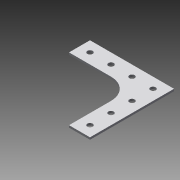
# Autodesk Inventor part: Gusset
Saved by Autodesk Inventor 2015 (Build 190159000, 159)
## iProperties
Created: 2015-01-30
Part Number: Gusset
Material: Generic
Document SubType Name: Modeling
Designer: chapale16
Density: 1 g/cm^3
Appearance: Default
Author: chapale16
Autodesk Inventor part; units mm, degrees
ref_plane "YZ Plane" through (0, 0, 0) normal (1, 0, 0) x (0, 1, 0)
ref_plane "XZ Plane" through (0, 0, 0) normal (0, 1, 0) x (-1, 0, 0)
ref_plane "XY Plane" through (0, 0, 0) normal (0, 0, 1) x (1, 0, 0)
sketch "Sketch1" plane through (0, 0, 0) normal (0, 1, 0) x (-1, 0, 0)
  line L0 (0, 0) -> (0, 101.6)
  line L1 (0, 101.6) -> (25.4, 101.6)
  line L2 (0, 0) -> (101.6, 0)
  line L3 (101.6, 0) -> (101.6, 25.4)
  line L4 (50.8, 25.4) -> (101.6, 25.4)
  line L5 (25.4, 50.8) -> (25.4, 101.6)
  arc A0 (25.4, 28.575) -> (28.575, 25.4) centre (28.575, 28.575) ccw
  arc A1 (25.4, 50.8) -> (50.8, 25.4) centre (50.8, 50.8) ccw
  dimension "d0" = 101.6
  dimension "d1" = 25.4
  dimension "d2" = 101.6
  dimension "d3" = 25.4
  dimension "d4" = 3.175
  dimension "d5" = 25.4
  constraints: 12 end point, 4 perpendicular, 4 point on circle, 4 tangent, 2 centre point, 2 point on line, 1 horizontal, 1 vertical
  measures "d0" distance of L0.start L0.end
  measures "d1" distance of L0.end L1.end
  measures "d2" distance of L0.start L2.end
  measures "d3" distance of L2.end L3.end
  measures "d4" radius of A0
  measures "d5" radius of A1
extrude "Extrusion1" add sketch "Sketch1" along normal blind 2.54
hole "Hole1" at (-12.7, 2.54, 12.7) direction (0, -1, 0) diameter 6.35 end through all
pattern_linear "Rectangular Pattern1" count 4 spacing 25.4 along (-1, 0, 0) of "Hole1"
pattern_linear "Rectangular Pattern2" count 4 spacing 25.4 along (0, 0, 1) of "Hole1"
body "Solid1"
